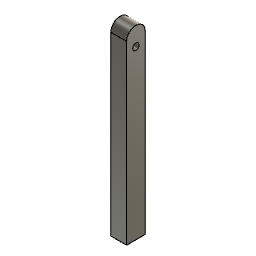
Final CAD v13 (Autodesk Fusion 360 archive; units mm, degrees)
design "零部件2123"
Autodesk Fusion 360 part; units mm, degrees
sketch "草图8" plane through (0, 0, 0) normal (0, 0, 1) x (1, 0, 0)
  line L0 (-8.5, 10) -> (8.5, 10)
  line L1 (8.5, 10) -> (8.5, -10)
  line L2 (8.5, -10) -> (-8.5, -10)
  line L3 (-8.5, -10) -> (-8.5, 10)
  line L4 (0, 1.75) -> (0, 22.5)
  line L5 (1.75, 0) -> (22.5, 0)
  dimension "d5" = 17
  dimension "d6" = 20
  constraint horizontal L0
  constraint vertical L1
  constraint horizontal L2
  constraint vertical L3
  constraint symmetric L1 L3 L4
  constraint symmetric L0 L2 L5
  measures "d5" distance of L0.start L0.end
  measures "d6" distance of L0.end L1.end
extrude "拉伸5" add sketch "草图8" along normal blind 200
fillet "圆角2" radius 10 2 edges at (0, -10, 200) (0, 10, 200)
sketch "草图10" plane through (8.5, 0, 0) normal (1, 0, 0) x (0, 1, 0)
  arc A0 (10, 190) -> (-10, 190) centre (0, 190) ccw
  line L0 (-10, 190) -> (-10, 0)
  line L1 (-10, 0) -> (10, 0)
  line L2 (10, 0) -> (10, 190)
  circle A1 centre (0, 180) radius 3.5
  dimension "d14" = 7
  dimension "d15" = 180
  constraint vertical origin A1.centre
  measures "d14" diameter of A1
  measures "d15" distance of origin A1.centre
extrude "拉伸6" cut sketch "草图10" against normal blind 175 contours A1
